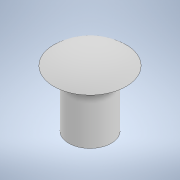
# Autodesk Inventor part: 0.188 in Rivet
Saved by Autodesk Inventor 2020 (Build 240168000, 168)
## iProperties
Created: 2020-01-14
Part Number: 0.188 in Rivet
Material: Generic
Document SubType Name: Modeling
Designer: aidan
Density: 1 g/cm^3
Appearance: Default
Author: aidan
Autodesk Inventor part; units mm, degrees
ref_plane "YZ Plane" through (0, 0, 0) normal (1, 0, 0) x (0, 1, 0)
ref_plane "XZ Plane" through (0, 0, 0) normal (0, 1, 0) x (-1, 0, 0)
ref_plane "XY Plane" through (0, 0, 0) normal (0, 0, 1) x (1, 0, 0)
sketch "Sketch1" plane through (0, 0, 0) normal (0, 0, 1) x (1, 0, 0)
  arc A0 (0, 2.4397) -> (-4.0481, 0.8203) centre (0, -3.4299) ccw
  line L0 (-4.0481, 0.8203) -> (-2.3813, 0.8203)
  line L1 (-2.3813, 0.8203) -> (-2.3812, -5.5297)
  line L2 (-2.3812, -5.5297) -> (0, -5.5297)
  line L3 (0, 8.0983) -> (0, -8.7405) construction
  line L4 (-7.3401, 2.4397) -> (11.6392, 2.4397) construction
  line L5 (0, 2.4397) -> (0, -5.5297)
  point P0 (0, 0)
  dimension "d0" = 2.3813
  dimension "d1" = 6.35
  dimension "d2" = 4.0481
  constraints: 12 end point, 4 point on line, 3 horizontal, 2 perpendicular, 2 point on circle, 1 centre point, 1 tangent, 1 vertical
  measures "d0" distance of L1.end L2.end
  measures "d1" distance of L0.end L1.end
  measures "d2" distance from line of L3 L0.start
revolve "Revolution1" add sketch "Sketch1" angle 360 about axis through (0, 8.0983, 0) along (0, -1, 0)
body "Solid1"
